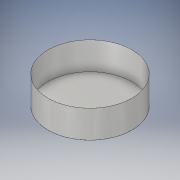
# Autodesk Inventor part: foil
Saved by Autodesk Inventor 2017 (Build 210142000, 142)
## iProperties
Created: 2017-06-10
Part Number: foil
Material: Aluminum 6061
Document SubType Name: Modeling
Designer: Blaire Weinberg
Density: 2.7 g/cm^3
Appearance: Aluminum - Polished
Author: Blaire Weinberg
Autodesk Inventor part; units mm, degrees
ref_plane "YZ Plane" through (0, 0, 0) normal (1, 0, 0) x (0, 1, 0)
ref_plane "XZ Plane" through (0, 0, 0) normal (0, 1, 0) x (-1, 0, 0)
ref_plane "XY Plane" through (0, 0, 0) normal (0, 0, 1) x (1, 0, 0)
sketch "Sketch1" plane through (0, 0, 0) normal (0, 1, 0) x (-1, 0, 0)
  circle A0 centre (0, -0.2393) radius 9.6603
  point P0 (0, 0)
  dimension "d0" = 19.3205
  constraints: 1 centre point
  measures "d0" diameter of A0
extrude "Extrusion1" add sketch "Sketch1" along normal blind 0.016
sketch "Sketch2" plane through (0, 0.016, -0.2393) normal (0, 1, 0) x (1, 0, 0)
  circle A0 centre (0, 0) radius 9.6603 projected
  circle A1 centre (0, 0) radius 9.6443
  point P0 (0, -0.2393)
  dimension "d3" = 0.016
  constraints: 1 centre point
  measures "d3" radial gap between concentric circles of A0 A1
extrude "Extrusion2" add sketch "Sketch2" along normal blind 6.35
body "Solid1"
